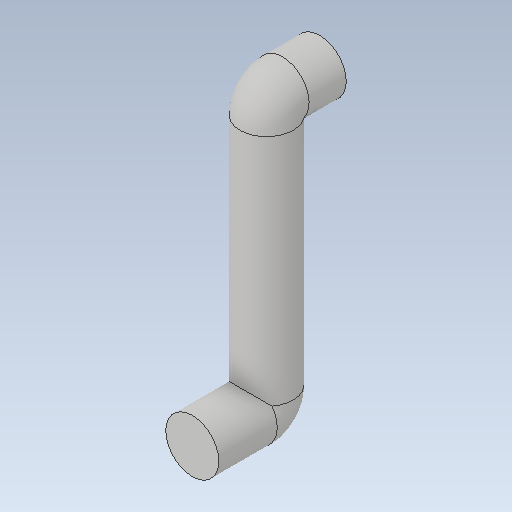
# Autodesk Inventor part: Exhaust
Saved by Autodesk Inventor 2020 (Build 240168000, 168)
## iProperties
Created: 2020-10-06
Part Number: Exhaust
Material: Generic
Document SubType Name: Modeling
Designer: nabee
Density: 1 g/cm^3
Appearance: Default
Author: nabee
Autodesk Inventor part; units mm, degrees
ref_plane "YZ Plane" through (0, 0, 0) normal (1, 0, 0) x (0, 1, 0)
ref_plane "XZ Plane" through (0, 0, 0) normal (0, 1, 0) x (-1, 0, 0)
ref_plane "XY Plane" through (0, 0, 0) normal (0, 0, 1) x (1, 0, 0)
ref_plane "Work Plane1" through (-527.9617, -1874.6232, 239.2901) normal (0, 0, 1) x (1, 0, 0)
sketch "Sketch7" plane through (-527.9617, -1874.6232, 239.2901) normal (0, 0, 1) x (1, 0, 0)
  circle A0 centre (0, 0) radius 25
  point P0 (527.9617, 1874.6232)
  dimension "d25" = 50
  constraints: 1 centre point
  measures "d25" diameter of A0
sketch3d "3D Sketch6"
  line L0 (-527.9617, -1874.6232, 239.2901) -> (-527.9617, -1874.6232, 274.2901)
  arc A0 (-527.9617, -1874.6232, 274.2901) -> (-527.9617, -1889.6232, 289.2901) centre (-527.9617, -1889.6232, 274.2901) ccw
  line L1 (-527.9617, -1889.6232, 289.2901) -> (-527.9617, -2109.6232, 289.2901)
  arc A1 (-527.9617, -2109.6232, 289.2901) -> (-527.9617, -2124.6232, 304.2901) centre (-527.9617, -2109.6232, 304.2901) ccw
  line L2 (-527.9617, -2124.6232, 304.2901) -> (-527.9617, -2124.6232, 359.2901)
  dimension "d22" = 50
  dimension "d23" = 250
  dimension "d24" = 70
  dimension "d26" = 15
  dimension "d27" = 15
sweep "Sweep1" add profiles "Sketch7" path "3D Sketch6"
body "Solid1"
